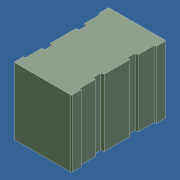
# Autodesk Inventor part: M20151ES1W03-switch
Saved by Autodesk Inventor 2014 (Build 180170000, 170)
## iProperties
Category: PARTsolutions
Created: 2013-12-29
Part Number: M20151ES1W03-switch
Catalog Web Link: www.cadenas.de
Description: Bushing Mount Miniature Toggles - Switch - Series M - Miniature Toggles
Document SubType Name: Modeling
Designer: PARTsolutions
Material: Generic
Density: 1 g/cm^3
Appearance: RGB(78,110,71)
NB: M20151ES1W03-switch
NN: Bushing Mount Miniature Toggles - Switch
NT: Series M - Miniature Toggles
NBSYN: $PN.-switch
LINA: M20151ES1W03-switch
PN: M20151ES1W03
SRS: M20
PLS: 1
CRCTSALG: '1','1 - ON/NONE/OFF','2','2 - ON/NONE/ON','3','3 - ON/OFF/ON','5','5 - ON/NONE/(ON)','8','8 - (ON)/OFF/(ON)','9','9 - ON/OFF/(ON)','4', '4 - ON/ON/ON','6','6 - (ON)/ON/(ON)','7','7 - ON/ON/(ON)'
CRCTS: 5
TGGL: 1
TGGLSALG: 'S', 'S - .413" (10.5mm) Bat','S2', 'S2 - .200" (5.08mm) Bat','S3', 'S3 - .256" (6.5mm) Bat','E', 'E - .450" (11.4mm) Flatted','E2', 'E2 - .256" (6.5mm) Flatted','E4', 'E4 - .840" (21.3mm) Flatted','Q', 'Q - .550" (14.0mm) Cone','Q2', 'Q2 - .640" (16.26mm) Cone','Q4', 'Q4 - .840" (21.3mm) Cone','C', 'C - .571" (14.5mm) Color Tipped Cone','D', 'D - .840" (21.3mm) Color Tipped Cone','K1', 'K1 - .370" (9.4mm) Paddle','K2', 'K2 - .559" (14.2mm) Paddle'
TGGLS: E
BSHNGALG: 'S1', 'S1 - .350" (8.9mm) Threaded with Keyway','S2', 'S2 - .350" (8.9mm) Smooth with Keyway','A1', 'A1 - .280" (7.1mm) Threaded with Keyway','A2', 'A2 - .280" (7.1mm) Smooth with Keyway','D1', 'D1 - .350" (8.9mm) Threaded with D Flat','D4' , 'D4 - 6mm .350" (8.9mm) Threaded with D Flat ' , 'S4', 'S4 - 6mm .350" (8.9mm) Threaded with Keyway'
BSHNG: S1
CMR: W
TRMNLSALG: '01','01 - Solder Lug','02','02 - Quick Connect','03','03 - .250" (6.35mm) Straight PC','05', '05 - .425" (10.8mm) Wirewrap','06', '06 - .750" (19.05mm) Wirewrap','07', '07 - .964" (24.5mm) Wirewrap','08', '08 - 1.062" (27.0mm) Wirewrap'
TRMNLS: 03
CPSALG: '','N/A'
CCLRALG: '','N/A'
WIDTH: 0.512
HEIGHT: 0.371
LENGTH: 0.311
A: 0.000
TRMNLNOH: 1.000
ROTALG: 0.262
ANG: 12.500
TRMNLOV: 3.000
LTRMNL: 0.073
POS: 0.000
KT: DUMMY
SUPPLIER: NKKSWITCHES
ARTICLENO: M20151ES1W03-switch
BOMINFO: M20151ES1W03-switch
CREATOR: CADENAS GmbH
PSOL_IDENT_0: {$CADENAS_DATA\23d-libs\nkkswitches\toggle\m\parts\m_bt_switch.prj},260 {VTYP=3D},{NB=M20151ES1W03-s
PSOL_IDENT_1: witch},{LINA=M20151ES1W03-switch},{NN=Bushing Mount Miniature Toggles - Switch},{DATE=28.05.2013 10:
PSOL_IDENT_2: 56:01},{GEOMDATE=28.05.2013 12:19:00},{VERSION=},{LINEID=10},{LINESUBID=-1},{WBVAR=PLS,CRCTS,TGGL,TG
PSOL_IDENT_3: GLS,BSHNG,CMR,TRMNLS,CPS,CCLR}  {NB=M20151ES1W03-switch},{LINA=M20151ES1W03-switch},{KT=DUMMY},{PN=M
PSOL_IDENT_4: 20151ES1W03},{SRS=M20},{PLS=1},{CRCTSALG='1','1 - ON/NONE/OFF','2','2 - ON/NONE/ON','3','3 - ON/OFF/
PSOL_IDENT_5: ON','5','5 - ON/NONE/(ON)','8','8 - (ON)/OFF/(ON)','9','9 - ON/OFF/(ON)','4', '4 - ON/ON/ON','6','6
PSOL_IDENT_6: - (ON)/ON/(ON)','7','7 - ON/ON/(ON)'},{CRCTS=5},{TGGL=1},{TGGLSALG='S', 'S - .413\" (10.5mm) Bat','S
PSOL_IDENT_7: 2', 'S2 - .200\" (5.08mm) Bat','S3', 'S3 - .256\" (6.5mm) Bat','E', 'E - .450\" (11.4mm) Flatted','E
PSOL_IDENT_8: 2', 'E2 - .256\" (6.5mm) Flatted','E4', 'E4 - .840\" (21.3mm) Flatted','Q', 'Q - .550\" (14.0mm) Con
PSOL_IDENT_9: e','Q2', 'Q2 - .640\" (16.26mm) Cone','Q4', 'Q4 - .840\" (21.3mm) Cone','C', 'C - .571\" (14.5mm) Co
PSOL_IDENT_10: lor Tipped Cone','D', 'D - .840\" (21.3mm) Color Tipped Cone','K1', 'K1 - .370\" (9.4mm) Paddle','K2
PSOL_IDENT_11: ', 'K2 - .559\" (14.2mm) Paddle'},{TGGLS=E},{BSHNGALG='S1', 'S1 - .350\" (8.9mm) Threaded with Keywa
PSOL_IDENT_12: y','S2', 'S2 - .350\" (8.9mm) Smooth with Keyway','A1', 'A1 - .280\" (7.1mm) Threaded with Keyway','
PSOL_IDENT_13: A2', 'A2 - .280\" (7.1mm) Smooth with Keyway','D1', 'D1 - .350\" (8.9mm) Threaded with D Flat','D4'
PSOL_IDENT_14: , 'D4 - 6mm .350\" (8.9mm) Threaded with D Flat ' , 'S4', 'S4 - 6mm .350\" (8.9mm) Threaded with Key
PSOL_IDENT_15: way'},{BSHNG=S1},{CMR=W},{TRMNLSALG='01','01 - Solder Lug','02','02 - Quick Connect','03','03 - .250
PSOL_IDENT_16: \" (6.35mm) Straight PC','05', '05 - .425\" (10.8mm) Wirewrap','06', '06 - .750\" (19.05mm) Wirewrap
PSOL_IDENT_17: ','07', '07 - .964\" (24.5mm) Wirewrap','08', '08 - 1.062\" (27.0mm) Wirewrap'},{TRMNLS=03},{CPSALG=
PSOL_IDENT_18: '','N/A'},{CPS=},{CPSPN=},{CCLRALG='','N/A'},{CCLR=},{DSH=},{WIDTH=0.512},{HEIGHT=0.371},{LENGTH=0.3
PSOL_IDENT_19: 11},{A=0},{TRMNLNOH=1},{ROTALG=0.2625},{ANG=12.5},{TRMNLOV=3},{LTRMNL=0.073},{POS=0}
Title: M20151ES1W03-switch
Author: Cadenas PARTsolutions
Comments: Series M - Miniature Toggles
Autodesk Inventor part; units mm, degrees
sketch "Sketch_2" plane through (0, -0.254, 0) normal (0, 1, 0) x (1, 0, 0)
  line L0 (-3.9497, -5.1435) -> (-3.9497, -6.3724)
  arc A0 (-3.9497, -6.3724) -> (-3.8197, -6.5024) centre (-3.8197, -6.3724) ccw
  line L1 (-3.8197, -6.5024) -> (3.8197, -6.5024)
  arc A1 (3.8197, -6.5024) -> (3.9497, -6.3724) centre (3.8197, -6.3724) ccw
  line L2 (3.9497, -6.3724) -> (3.9497, -5.1435)
  line L3 (3.9497, -5.1435) -> (3.6957, -5.1435)
  line L4 (3.6957, -5.1435) -> (3.6957, -2.9397)
  line L5 (3.6957, -2.9397) -> (3.3147, -2.8725)
  line L6 (3.3147, -2.8725) -> (3.3147, -1.8265)
  line L7 (3.3147, -1.8265) -> (3.6957, -1.7593)
  line L8 (3.6957, -1.7593) -> (3.6957, 1.7593)
  line L9 (3.6957, 1.7593) -> (3.3147, 1.8265)
  line L10 (3.3147, 1.8265) -> (3.3147, 2.8725)
  line L11 (3.3147, 2.8725) -> (3.6957, 2.9397)
  line L12 (3.6957, 2.9397) -> (3.6957, 5.1435)
  line L13 (3.6957, 5.1435) -> (3.9497, 5.1435)
  line L14 (3.9497, 5.1435) -> (3.9497, 6.3724)
  arc A2 (3.9497, 6.3724) -> (3.8197, 6.5024) centre (3.8197, 6.3724) ccw
  line L15 (3.8197, 6.5024) -> (-3.8197, 6.5024)
  arc A3 (-3.8197, 6.5024) -> (-3.9497, 6.3724) centre (-3.8197, 6.3724) ccw
  line L16 (-3.9497, 6.3724) -> (-3.9497, 5.1435)
  line L17 (-3.9497, 5.1435) -> (-3.6957, 5.1435)
  line L18 (-3.6957, 5.1435) -> (-3.6957, 2.9397)
  line L19 (-3.6957, 2.9397) -> (-3.3147, 2.8725)
  line L20 (-3.3147, 2.8725) -> (-3.3147, 1.8265)
  line L21 (-3.3147, 1.8265) -> (-3.6957, 1.7593)
  line L22 (-3.6957, 1.7593) -> (-3.6957, -1.7593)
  line L23 (-3.6957, -1.7593) -> (-3.3147, -1.8265)
  line L24 (-3.3147, -1.8265) -> (-3.3147, -2.8725)
  line L25 (-3.3147, -2.8725) -> (-3.6957, -2.9397)
  line L26 (-3.6957, -2.9397) -> (-3.6957, -5.1435)
  line L27 (-3.6957, -5.1435) -> (-3.9497, -5.1435)
  constraints: 56 end point, 8 point on circle, 4 centre point
extrude "Extrusion1" add sketch "Sketch_2" against normal blind 9.1694
sketch "Sketch_1" plane through (0, -9.4234, 0) normal (0, 1, 0) x (1, 0, 0)
  line L0 (-3.1877, 6.1184) -> (-3.1877, -6.1184)
  arc A0 (-3.1877, -6.1184) -> (-3.0577, -6.2484) centre (-3.0577, -6.1184) ccw
  line L1 (-3.0577, -6.2484) -> (3.0577, -6.2484)
  arc A1 (3.0577, -6.2484) -> (3.1877, -6.1184) centre (3.0577, -6.1184) ccw
  line L2 (3.1877, -6.1184) -> (3.1877, 6.1184)
  arc A2 (3.1877, 6.1184) -> (3.0577, 6.2484) centre (3.0577, 6.1184) ccw
  line L3 (3.0577, 6.2484) -> (-3.0577, 6.2484)
  arc A3 (-3.0577, 6.2484) -> (-3.1877, 6.1184) centre (-3.0577, 6.1184) ccw
  constraints: 8 end point, 8 point on circle, 4 centre point
extrude "Extrusion2" cut sketch "Sketch_1" along normal blind 0.0254
sketch "Sketch_7" plane through (0, -9.4234, 0) normal (0, 1, 0) x (1, 0, 0)
  line L0 (-0.9271, 5.0927) -> (-0.9271, 4.3053)
  line L1 (-0.9271, 4.3053) -> (0.9271, 4.3053)
  line L2 (0.9271, 4.3053) -> (0.9271, 5.0927)
  line L3 (0.9271, 5.0927) -> (-0.9271, 5.0927)
  constraints: 8 end point
extrude "Extrusion3" cut sketch "Sketch_7" along normal blind 0.254
pattern_linear "Rectangular Pattern1" count 3 spacing 4.699 along (0, 0, 1) of "Extrusion3"
ref_plane "rot_XY" through (0, 6.6675, 0) normal (1, 0, 0) x (0, 0, -1)
ref_plane "rot_YZ" through (0, 6.6675, 0) normal (0, 0, -1) x (0, 1, 0)
ref_plane "rot_ZX" through (0, 6.6675, 0) normal (0, 1, 0) x (1, 0, 0)
ref_plane "to_cover_XY" through (0, -0.254, 0) normal (0, 1, 0) x (1, 0, 0)
ref_plane "to_cover_YZ" through (0, -0.254, 0) normal (1, 0, 0) x (0, 0, -1)
ref_plane "to_cover_ZX" through (0, -0.254, 0) normal (0, 0, -1) x (0, 1, 0)
ref_plane "to_terminals_XY" through (0, -9.4234, 0) normal (0, 1, 0) x (1, 0, 0)
ref_plane "to_terminals_YZ" through (0, -9.4234, 0) normal (1, 0, 0) x (0, 0, -1)
ref_plane "to_terminals_ZX" through (0, -9.4234, 0) normal (0, 0, -1) x (0, 1, 0)
body "Solid1"
